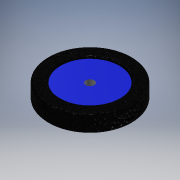
# Autodesk Inventor part: wiel
Saved by Autodesk Inventor 2017 (Build 210142000, 142)
## iProperties
Created: 2017-02-19
Part Number: wiel
Material: Generic
Document SubType Name: Modeling
Designer: user
Density: 1 g/cm^3
Appearance: Default
Author: user
Autodesk Inventor part; units mm, degrees
ref_plane "YZ Plane" through (0, 0, 0) normal (1, 0, 0) x (0, 1, 0)
ref_plane "XZ Plane" through (0, 0, 0) normal (0, 1, 0) x (-1, 0, 0)
ref_plane "XY Plane" through (0, 0, 0) normal (0, 0, 1) x (1, 0, 0)
sketch "Sketch1" plane through (0, 0, 0) normal (1, 0, 0) x (0, 1, 0)
  line L0 (0, 280.159) -> (0, -280.159)
  line L1 (0, 15) -> (70, 15)
  line L2 (70, 15) -> (70, 15)
  line L3 (75, 20) -> (95, 20)
  line L4 (100, 15) -> (100, -15)
  line L5 (95, -20) -> (75, -20)
  line L6 (70, -15) -> (70, -15)
  line L7 (70, -15) -> (0, -15)
  line L8 (0, 15) -> (0, -15)
  line L9 (0, 0) -> (100, 0)
  arc A0 (98, -20) -> (100, -18) centre (98, -18) ccw
  arc A1 (95, -20) -> (100, -15) centre (95, -15) ccw
  arc A2 (100, 15) -> (95, 20) centre (95, 15) ccw
  arc A3 (75, 20) -> (70, 15) centre (75, 15) ccw
  arc A4 (70, -15) -> (75, -20) centre (75, -15) ccw
  line L10 (10, 15) -> (10, -15)
  point P0 (100, 20)
  point P1 (100, -20)
  point P2 (70, -20)
  dimension "d0" = 560.3179
  dimension "d1" = 40
  dimension "d2" = 30
  dimension "d3" = 30
  dimension "d4" = 200
  dimension "d5" = 2
  dimension "d6" = 5
  dimension "d7" = 20
  constraints: 22 end point, 14 point on line, 10 point on circle, 10 tangent, 8 perpendicular, 5 centre point, 3 equal radius, 2 midpoint, 1 coincident, 1 horizontal, 1 horizontal alignment, 1 vertical, 2 other
  measures "d0" distance of L0.start L0.end
  measures "d1" distance of point (100, 20) point (100, -20)
  measures "d2" distance between parallel lines of L1 L7
  measures "d3" distance of point (100, -20) point (70, -20)
  measures "d4" diameter of L4 L0
  measures "d5" radius of A0
  measures "d6" radius of A1
  measures "d7" diameter of L10 L0
revolve "Revolution1" add sketch "Sketch1" angle 360 about axis through (0, 0, 280.159) along (0, 0, -1) contours L1 A3 L3 A2 L4 L9 L10 | L9 L4 A1 L5 A4 L7 L10
body "Solid1"
